skadis_nut_coupon (Autodesk Fusion 360 design; units mm, degrees)
part number: 2026-09-06-14-40-16-018
Autodesk Fusion 360 part; units mm, degrees
sketch "Plate" plane through (0, 0, 0) normal (0, 1, 0) x (1, 0, 0)
  line L0 (0, 0) -> (11, 0)
  line L1 (11, 0) -> (11, -20)
  line L2 (11, -20) -> (0, -20)
  line L3 (0, -20) -> (0, 0)
  dimension "d102" = 11
  dimension "d103" = 20
  constraint coincident L0.start L3.end
  constraint horizontal L0
  constraint horizontal L2
  constraint vertical L1
  constraint vertical L3
  measures "d102" horizontal distance of L0.start L1.end
  measures "d103" vertical distance of L0.start L1.end
extrude "Plate (1)" add sketch "Plate" along normal mid plane 33 from surface at 4.5
sketch "Screw hole" plane through (0, 0, 0) normal (0, 1, 0) x (1, 0, 0)
  line L0 (-1, -7.6) -> (12, -7.6)
  line L1 (12, -7.6) -> (12, -12.4)
  line L2 (12, -12.4) -> (-1, -12.4)
  line L3 (-1, -12.4) -> (-1, -7.6)
  dimension "d107" = 12
  dimension "d108" = 7.6
  dimension "d109" = 13
  dimension "d110" = 4.8
  constraint horizontal L0
  constraint horizontal L2
  constraint vertical L1
  constraint vertical L3
  measures "d107" horizontal distance of origin L0.end
  measures "d108" vertical distance of origin L0.end
  measures "d109" horizontal distance of L0.start L0.end
  measures "d110" vertical distance of L0.end L1.end
extrude "Screw hole (1)" cut sketch "Screw hole" along normal mid plane 16.8 from surface at 7.52
sketch "Nut cavity" plane through (0, 0, 0) normal (0, 1, 0) x (1, 0, 0)
  line L0 (3.6, -6.3) -> (7, -6.3)
  line L1 (7, -6.3) -> (7, -13.7)
  line L2 (7, -13.7) -> (3.6, -13.7)
  line L3 (3.6, -13.7) -> (3.6, -6.3)
  dimension "d114" = 7
  dimension "d115" = 6.3
  dimension "d116" = 3.4
  dimension "d117" = 7.4
  constraint horizontal L0
  constraint horizontal L2
  constraint vertical L1
  constraint vertical L3
  measures "d114" horizontal distance of origin L0.end
  measures "d115" vertical distance of origin L0.end
  measures "d116" horizontal distance of L0.start L0.end
  measures "d117" vertical distance of L0.end L1.end
extrude "Nut cavity (1)" cut sketch "Nut cavity" along normal mid plane 30.22 from surface at 2.11
equation "bracketWidth = 24.0 mm" comment "bracket width across the upright"
equation "plateHeight = 20.0 mm" comment "plate height"
equation "plateInboardExtension = 9.0 mm" comment "extra plate toward the desk centre, where the channel reaches"
equation "boardThickness = 6.0 mm" comment "measured SKADIS panel thickness"
equation "screwLength = 15.0 mm" comment "measured decorative M4 screw"
equation "screwDiameter = 4.0 mm" comment "M4 shank"
equation "screwClearance = 0.8 mm" comment "slack around the shank"
equation "screwTipClearance = 2.0 mm" comment "tip stops this short of the plate's back face"
equation "screwSlotWidth = screwDiameter + screwClearance" comment "screw relief slot height"
equation "nutAcrossFlats = 7.0 mm" comment "M4 square nut across flats"
equation "nutThickness = 3.0 mm" comment "M4 square nut thickness"
equation "nutChannelClearance = 0.4 mm" comment "slack around the nut in its channel"
equation "nutChannelHeight = nutAcrossFlats + nutChannelClearance" comment "channel height; under the nut's diagonal so it cannot turn"
equation "plateThickness = screwLength - boardThickness + screwTipClearance" comment "derived: deep enough to swallow the screw"
equation "mountTravel = 12.0 mm" comment "left-right adjustment"
equation "nutChannelLength = mountTravel + nutAcrossFlats + nutChannelClearance" comment "channel length along the plate"
equation "screwSlotLength = mountTravel + screwSlotWidth" comment "relief slot length along the plate"
equation "topMountZ = 10.0 mm" comment "top channel centre"
equation "mountOffsetY = 7.52 mm" comment "channel centre on the board's grid"
equation "slotOvershoot = 1.0 mm" comment "cuts reach past the faces they cut"
equation "nutCavityClearance = 0.4 mm" comment "slack across the nut's thickness"
equation "nutWallThickness = 4.0 mm" comment "wall in front of the nut; the screw pulls the nut against it"
equation "nutCavityDepth = nutThickness + nutCavityClearance" comment "cavity depth"
equation "d102 = plateThickness"
equation "d103 = plateHeight"
equation "d104 = plateInboardExtension / 2"
equation "d105 = bracketWidth + plateInboardExtension"
equation "d107 = plateThickness + slotOvershoot"
equation "d108 = topMountZ - screwSlotWidth / 2"
equation "d109 = plateThickness + 2 * slotOvershoot"
equation "d110 = screwSlotWidth"
equation "d111 = mountOffsetY"
equation "d112 = screwSlotLength"
equation "d114 = plateThickness - nutWallThickness"
equation "d115 = topMountZ - nutChannelHeight / 2"
equation "d116 = nutCavityDepth"
equation "d117 = nutChannelHeight"
equation "d118 = ( mountOffsetY + nutChannelLength / 2 - bracketWidth / 2 - slotOvershoot ) / 2"
equation "d119 = mountOffsetY + nutChannelLength / 2 + bracketWidth / 2 + slotOvershoot"
named bodies: "skadis_nut_coupon"
